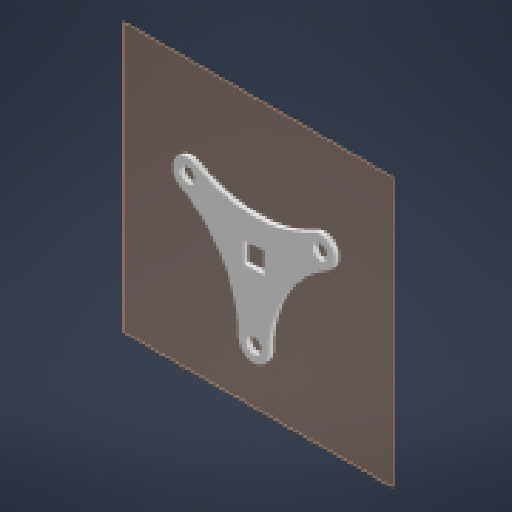
# Autodesk Inventor part: 3in flex wheel holder
Saved by Autodesk Inventor 2025.4 (Build 294407000, 407)
## iProperties
Created: 2026-01-22
Part Number: 3in flex wheel holder
Material: Generic
Document SubType Name: Modeling
Designer: shaun
Density: 1 g/cm^3
Appearance: Default
Author: shaun
Autodesk Inventor part; units mm, degrees
ref_plane "YZ Plane" through (0, 0, 0) normal (1, 0, 0) x (0, 1, 0)
ref_plane "XZ Plane" through (0, 0, 0) normal (0, 1, 0) x (-1, 0, 0)
ref_plane "XY Plane" through (0, 0, 0) normal (0, 0, 1) x (1, 0, 0)
ref_plane "Work Plane1" through (0, 0, 0) normal (0, 0, 1) x (1, 0, 0)
sketch "Sketch1" plane through (0, 0, 0) normal (0, 0, 1) x (1, 0, 0)
  circle A0 centre (0, -23.8125) radius 2.1526 construction
  circle A1 centre (20.6222, 11.9063) radius 2.1526 construction
  circle A2 centre (-20.6222, 11.9062) radius 2.1526 construction
  line L0 (2.7178, 3.2258) -> (-2.7178, 3.2258)
  line L1 (-3.2258, 2.7178) -> (-3.2258, -2.7178)
  line L2 (-2.7178, -3.2258) -> (2.7178, -3.2258)
  line L3 (3.2258, -2.7178) -> (3.2258, 2.7178)
  line L4 (3.2258, 3.2258) -> (-3.2258, -3.2258) construction
  line L5 (-3.2258, 3.2258) -> (3.2258, -3.2258) construction
  arc A3 (2.7178, -3.2258) -> (3.2258, -2.7178) centre (2.7178, -2.7178) ccw
  arc A4 (-3.2258, -2.7178) -> (-2.7178, -3.2258) centre (-2.7178, -2.7178) ccw
  arc A5 (-2.7178, 3.2258) -> (-3.2258, 2.7178) centre (-2.7178, 2.7178) ccw
  arc A6 (3.2258, 2.7178) -> (2.7178, 3.2258) centre (2.7178, 2.7178) ccw
  circle A7 centre (0, 0) radius 11.1125
  circle A8 centre (0, -23.8125) radius 4.7625
  circle A9 centre (-20.6222, 11.9062) radius 4.7625
  circle A10 centre (20.6222, 11.9063) radius 4.7625
  arc A11 (22.9921, 7.7752) -> (4.7625, -23.7993) centre (41.0481, -23.6991) ccw
  arc A12 (-18.2296, 16.0241) -> (18.2296, 16.0241) centre (0, 47.3982) ccw
  arc A13 (-4.7625, -23.7993) -> (-22.9921, 7.7752) centre (-41.0481, -23.6991) ccw
  circle A14 centre (0, -23.8125) radius 2.2479
  circle A15 centre (20.6222, 11.9062) radius 2.2479
  circle A16 centre (-20.6222, 11.9063) radius 2.2479
  point P0 (18.2296, 16.0241)
  point P1 (-18.2296, 16.0241)
  point P2 (-22.9921, 7.7752)
  point P3 (-4.7625, -23.7993)
  dimension "d3" = 9.525
  dimension "d0" = 0.508
  dimension "d1" = 6.4516
  dimension "d2" = 22.225
  dimension "d6" = 360
  dimension "d8" = 4.4958
  dimension "d11" = 360
  constraints: 14 point on circle, 12 centre point, 12 end point, 9 tangent, 8 point on line, 5 coincident, 3 equal radius, 2 midpoint, 2 parallel, 2 perpendicular, 1 horizontal, 29 other
  measures "d0" radius of A3
  measures "d1" distance between parallel lines of L1 L3
  measures "d2" diameter of A7
  measures "d8" diameter of A14
extrude "Extrusion1" add sketch "Sketch1" along normal blind 1.5
body "Solid1"
